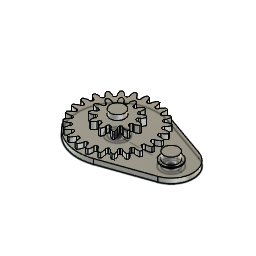
spur_gear_v2 (Autodesk Fusion 360 design; units mm, degrees)
part number: 2025-08-28-16-30-15-066
description: Spur Gear; Module: 3.0; Num Teeth: 24; Pressure Angle: 20.0; Backlash: 0.25 mm
part number: 2025-08-28-16-46-57-716
description: Spur Gear; Module: 3.0; Num Teeth: 12; Pressure Angle: 20.0; Backlash: 0.25 mm
part number: 2025-08-28-16-47-23-032
Autodesk Fusion 360 part; units mm, degrees
sketch "Sketch1" plane through (0, 0, 0) normal (0, 0, 1) x (1, 0, 0) in component "Spur Gear (24 teeth)"
  circle A0 centre (0, 0) radius 32.3492
  circle A1 centre (0, 0) radius 7.5
extrude "Extrude1" add sketch "Sketch1" along normal blind 5 makes body 1 in component "Spur Gear (24 teeth)"
sketch "Sketch2" plane through (0, 0, 0) normal (0, 0, 1) x (1, 0, 0) in component "Spur Gear (24 teeth)"
  spline S0 degree 5 poles (33.7244, -2.6568) (33.7396, -2.658) (33.77, -2.66) (33.8155, -2.6619) (33.8763, -2.6622) (33.9524, -2.6596) (34.0285, -2.6548) (34.1046, -2.6488) (34.1808, -2.642) (34.257, -2.6347) (34.3333, -2.6269) (34.4095, -2.6185) (34.4857, -2.6091) (34.5619, -2.5987) (34.6382, -2.5873) (34.7144, -2.5749) (34.7906, -2.5617) (34.8667, -2.5478) (34.9429, -2.5333) (35.019, -2.5183) (35.0952, -2.5027) (35.1712, -2.4864) (35.2473, -2.4696) (35.3234, -2.4521) (35.3994, -2.434) (35.4753, -2.4152) (35.5513, -2.3959) (35.6272, -2.376) (35.7031, -2.3556) (35.7789, -2.3347) (35.8547, -2.3132) (35.9304, -2.2912) (36.0062, -2.2688) (36.0818, -2.2458) (36.1575, -2.2223) (36.233, -2.1983) (36.3086, -2.1738) (36.384, -2.1488) (36.4595, -2.1233) (36.5349, -2.0974) (36.6102, -2.071) (36.6855, -2.0442) (36.7607, -2.0169) (36.8358, -1.9892) (36.911, -1.961) (36.986, -1.9324) (37.061, -1.9033) (37.1359, -1.8738) (37.2108, -1.8439) (37.2856, -1.8135) (37.3604, -1.7828) (37.435, -1.7516) (37.5097, -1.72) (37.5842, -1.688) (37.6587, -1.6556) (37.7331, -1.6227) (37.8075, -1.5895) (37.8818, -1.5559) (37.956, -1.5219) (38.0301, -1.4875) (38.1042, -1.4527) (38.1782, -1.4175) (38.2521, -1.3819) (38.3259, -1.346) (38.3997, -1.3096) (38.4734, -1.2729) (38.547, -1.2358) (38.6206, -1.1984) (38.694, -1.1606) (38.7674, -1.1224) (38.8407, -1.0838) (38.8993, -1.0527) (38.9432, -1.0292) (38.9724, -1.0134) (38.987, -1.0055) knots 0 0 0 0 0 0 0.01428571 0.02857143 0.04285714 0.05714286 0.07142857 0.08571429 0.1 0.11428571 0.12857143 0.14285714 0.15714286 0.17142857 0.18571429 0.2 0.21428571 0.22857143 0.24285714 0.25714286 0.27142857 0.28571429 0.3 0.31428571 0.32857143 0.34285714 0.35714286 0.37142857 0.38571429 0.4 0.41428571 0.42857143 0.44285714 0.45714286 0.47142857 0.48571429 0.5 0.51428571 0.52857143 0.54285714 0.55714286 0.57142857 0.58571429 0.6 0.61428571 0.62857143 0.64285714 0.65714286 0.67142857 0.68571429 0.7 0.71428571 0.72857143 0.74285714 0.75714286 0.77142857 0.78571429 0.8 0.81428571 0.82857143 0.84285714 0.85714286 0.87142857 0.88571429 0.9 0.91428571 0.92857143 0.94285714 0.95714286 0.97142857 0.98571429 1 1 1 1 1 1
  spline S1 degree 5 poles (33.7244, 2.6568) (33.7396, 2.658) (33.77, 2.66) (33.8155, 2.6619) (33.8763, 2.6622) (33.9524, 2.6596) (34.0285, 2.6548) (34.1046, 2.6488) (34.1808, 2.642) (34.257, 2.6347) (34.3333, 2.6269) (34.4095, 2.6185) (34.4857, 2.6091) (34.5619, 2.5987) (34.6382, 2.5873) (34.7144, 2.5749) (34.7906, 2.5617) (34.8667, 2.5478) (34.9429, 2.5333) (35.019, 2.5183) (35.0952, 2.5027) (35.1712, 2.4864) (35.2473, 2.4696) (35.3234, 2.4521) (35.3994, 2.434) (35.4753, 2.4152) (35.5513, 2.3959) (35.6272, 2.376) (35.7031, 2.3556) (35.7789, 2.3347) (35.8547, 2.3132) (35.9304, 2.2912) (36.0062, 2.2688) (36.0818, 2.2458) (36.1575, 2.2223) (36.233, 2.1983) (36.3086, 2.1738) (36.384, 2.1488) (36.4595, 2.1233) (36.5349, 2.0974) (36.6102, 2.071) (36.6855, 2.0442) (36.7607, 2.0169) (36.8358, 1.9892) (36.911, 1.961) (36.986, 1.9324) (37.061, 1.9033) (37.1359, 1.8738) (37.2108, 1.8439) (37.2856, 1.8135) (37.3604, 1.7828) (37.435, 1.7516) (37.5097, 1.72) (37.5842, 1.688) (37.6587, 1.6556) (37.7331, 1.6227) (37.8075, 1.5895) (37.8818, 1.5559) (37.956, 1.5219) (38.0301, 1.4875) (38.1042, 1.4527) (38.1782, 1.4175) (38.2521, 1.3819) (38.3259, 1.346) (38.3997, 1.3096) (38.4734, 1.2729) (38.547, 1.2358) (38.6206, 1.1984) (38.694, 1.1606) (38.7674, 1.1224) (38.8407, 1.0838) (38.8993, 1.0527) (38.9432, 1.0292) (38.9724, 1.0134) (38.987, 1.0055) knots 0 0 0 0 0 0 0.01428571 0.02857143 0.04285714 0.05714286 0.07142857 0.08571429 0.1 0.11428571 0.12857143 0.14285714 0.15714286 0.17142857 0.18571429 0.2 0.21428571 0.22857143 0.24285714 0.25714286 0.27142857 0.28571429 0.3 0.31428571 0.32857143 0.34285714 0.35714286 0.37142857 0.38571429 0.4 0.41428571 0.42857143 0.44285714 0.45714286 0.47142857 0.48571429 0.5 0.51428571 0.52857143 0.54285714 0.55714286 0.57142857 0.58571429 0.6 0.61428571 0.62857143 0.64285714 0.65714286 0.67142857 0.68571429 0.7 0.71428571 0.72857143 0.74285714 0.75714286 0.77142857 0.78571429 0.8 0.81428571 0.82857143 0.84285714 0.85714286 0.87142857 0.88571429 0.9 0.91428571 0.92857143 0.94285714 0.95714286 0.97142857 0.98571429 1 1 1 1 1 1
  arc A0 (38.987, -1.0055) -> (38.987, 1.0055) centre (0, 0) ccw
  line L0 (32.2393, -2.5406) -> (33.7244, -2.6568)
  line L1 (32.2393, 2.5406) -> (33.7244, 2.6568)
  line L2 (32.2393, -2.5406) -> (32.2393, 2.5406)
  point P0 (34.0955, -2.6493)
  point P1 (34.4689, -2.611)
  point P2 (34.8437, -2.552)
  point P3 (35.2195, -2.4757)
  point P4 (35.596, -2.3841)
  point P5 (35.973, -2.2785)
  point P6 (36.3504, -2.1599)
  point P7 (36.7278, -2.0288)
  point P8 (37.1053, -1.8858)
  point P9 (37.4826, -1.7314)
  point P10 (37.8595, -1.5659)
  point P11 (38.236, -1.3896)
  point P12 (38.6119, -1.2027)
  point P13 (34.0955, 2.6493)
  point P14 (34.4689, 2.611)
  point P15 (34.8437, 2.552)
  point P16 (35.2195, 2.4757)
  point P17 (35.596, 2.3841)
  point P18 (35.973, 2.2785)
  point P19 (36.3504, 2.1599)
  point P20 (36.7278, 2.0288)
  point P21 (37.1053, 1.8858)
  point P22 (37.4826, 1.7314)
  point P23 (37.8595, 1.5659)
  point P24 (38.236, 1.3896)
  point P25 (38.6119, 1.2027)
extrude "Extrude2" add sketch "Sketch2" along normal blind 5 bodies 1 in component "Spur Gear (24 teeth)"
fillet "Fillet1" radius 1.58 2 edges at (32.2492, -2.5414, 2.5) (32.2492, 2.5414, 2.5) on bodies 1 in component "Spur Gear (24 teeth)"
pattern_circular "C-Pattern1" count 24 over 360 about axis through (0, 0, 0) along (0, 0, 1) of "Extrude2", "Fillet1" in component "Spur Gear (24 teeth)"
sketch "Sketch3" plane through (0, 0, 0) normal (0, 0, 1) x (1, 0, 0) in component "Spur Gear (24 teeth)"
  circle A0 centre (0, 0) radius 36 construction
sketch "Sketch1 (2)" plane through (0, 0, 0) normal (0, 0, 1) x (1, 0, 0) in component "Spur Gear (12 teeth)"
  circle A0 centre (0, 0) radius 14.3492
  circle A1 centre (0, 0) radius 7.5
extrude "Extrude1'" add sketch "Sketch1 (2)" along normal blind 5 separate body makes body 2 in component "Spur Gear (12 teeth)"
sketch "Sketch2 (2)" plane through (0, 0, 0) normal (0, 0, 1) x (1, 0, 0) in component "Spur Gear (12 teeth)"
  spline S0 degree 5 poles (16.7434, -2.3993) (16.7555, -2.4011) (16.7797, -2.4041) (16.816, -2.4076) (16.8646, -2.4099) (16.9256, -2.4099) (16.9867, -2.4077) (17.048, -2.4042) (17.1093, -2.3999) (17.1707, -2.3952) (17.2321, -2.3899) (17.2936, -2.3839) (17.3551, -2.377) (17.4166, -2.369) (17.4782, -2.3599) (17.5398, -2.3498) (17.6015, -2.3389) (17.6631, -2.3273) (17.7248, -2.3151) (17.7864, -2.3023) (17.8481, -2.2889) (17.9097, -2.2748) (17.9713, -2.2601) (18.0329, -2.2447) (18.0945, -2.2286) (18.1561, -2.2119) (18.2176, -2.1946) (18.2792, -2.1767) (18.3407, -2.1582) (18.4021, -2.1392) (18.4635, -2.1196) (18.5249, -2.0995) (18.5863, -2.0788) (18.6476, -2.0576) (18.7089, -2.0358) (18.7701, -2.0135) (18.8312, -1.9906) (18.8923, -1.9673) (18.9534, -1.9434) (19.0144, -1.9191) (19.0753, -1.8942) (19.1362, -1.8689) (19.197, -1.8431) (19.2578, -1.8167) (19.3185, -1.7899) (19.3791, -1.7626) (19.4396, -1.7349) (19.5001, -1.7066) (19.5605, -1.6779) (19.6208, -1.6488) (19.681, -1.6192) (19.7412, -1.5891) (19.8013, -1.5586) (19.8612, -1.5276) (19.9211, -1.4962) (19.981, -1.4644) (20.0407, -1.4321) (20.1003, -1.3994) (20.1598, -1.3662) (20.2193, -1.3327) (20.2786, -1.2986) (20.3379, -1.2642) (20.397, -1.2294) (20.456, -1.1941) (20.515, -1.1584) (20.5738, -1.1223) (20.6325, -1.0858) (20.6911, -1.0489) (20.7496, -1.0116) (20.808, -0.9739) (20.8663, -0.9357) (20.9128, -0.9049) (20.9477, -0.8816) (20.9709, -0.866) (20.9825, -0.8582) knots 0 0 0 0 0 0 0.01428571 0.02857143 0.04285714 0.05714286 0.07142857 0.08571429 0.1 0.11428571 0.12857143 0.14285714 0.15714286 0.17142857 0.18571429 0.2 0.21428571 0.22857143 0.24285714 0.25714286 0.27142857 0.28571429 0.3 0.31428571 0.32857143 0.34285714 0.35714286 0.37142857 0.38571429 0.4 0.41428571 0.42857143 0.44285714 0.45714286 0.47142857 0.48571429 0.5 0.51428571 0.52857143 0.54285714 0.55714286 0.57142857 0.58571429 0.6 0.61428571 0.62857143 0.64285714 0.65714286 0.67142857 0.68571429 0.7 0.71428571 0.72857143 0.74285714 0.75714286 0.77142857 0.78571429 0.8 0.81428571 0.82857143 0.84285714 0.85714286 0.87142857 0.88571429 0.9 0.91428571 0.92857143 0.94285714 0.95714286 0.97142857 0.98571429 1 1 1 1 1 1
  spline S1 degree 5 poles (16.7434, 2.3993) (16.7555, 2.4011) (16.7797, 2.4041) (16.816, 2.4076) (16.8646, 2.4099) (16.9256, 2.4099) (16.9867, 2.4077) (17.048, 2.4042) (17.1093, 2.3999) (17.1707, 2.3952) (17.2321, 2.3899) (17.2936, 2.3839) (17.3551, 2.377) (17.4166, 2.369) (17.4782, 2.3599) (17.5398, 2.3498) (17.6015, 2.3389) (17.6631, 2.3273) (17.7248, 2.3151) (17.7864, 2.3023) (17.8481, 2.2889) (17.9097, 2.2748) (17.9713, 2.2601) (18.0329, 2.2447) (18.0945, 2.2286) (18.1561, 2.2119) (18.2176, 2.1946) (18.2792, 2.1767) (18.3407, 2.1582) (18.4021, 2.1392) (18.4635, 2.1196) (18.5249, 2.0995) (18.5863, 2.0788) (18.6476, 2.0576) (18.7089, 2.0358) (18.7701, 2.0135) (18.8312, 1.9906) (18.8923, 1.9673) (18.9534, 1.9434) (19.0144, 1.9191) (19.0753, 1.8942) (19.1362, 1.8689) (19.197, 1.8431) (19.2578, 1.8167) (19.3185, 1.7899) (19.3791, 1.7626) (19.4396, 1.7349) (19.5001, 1.7066) (19.5605, 1.6779) (19.6208, 1.6488) (19.681, 1.6192) (19.7412, 1.5891) (19.8013, 1.5586) (19.8612, 1.5276) (19.9211, 1.4962) (19.981, 1.4644) (20.0407, 1.4321) (20.1003, 1.3994) (20.1598, 1.3662) (20.2193, 1.3327) (20.2786, 1.2986) (20.3379, 1.2642) (20.397, 1.2294) (20.456, 1.1941) (20.515, 1.1584) (20.5738, 1.1223) (20.6325, 1.0858) (20.6911, 1.0489) (20.7496, 1.0116) (20.808, 0.9739) (20.8663, 0.9357) (20.9128, 0.9049) (20.9477, 0.8816) (20.9709, 0.866) (20.9825, 0.8582) knots 0 0 0 0 0 0 0.01428571 0.02857143 0.04285714 0.05714286 0.07142857 0.08571429 0.1 0.11428571 0.12857143 0.14285714 0.15714286 0.17142857 0.18571429 0.2 0.21428571 0.22857143 0.24285714 0.25714286 0.27142857 0.28571429 0.3 0.31428571 0.32857143 0.34285714 0.35714286 0.37142857 0.38571429 0.4 0.41428571 0.42857143 0.44285714 0.45714286 0.47142857 0.48571429 0.5 0.51428571 0.52857143 0.54285714 0.55714286 0.57142857 0.58571429 0.6 0.61428571 0.62857143 0.64285714 0.65714286 0.67142857 0.68571429 0.7 0.71428571 0.72857143 0.74285714 0.75714286 0.77142857 0.78571429 0.8 0.81428571 0.82857143 0.84285714 0.85714286 0.87142857 0.88571429 0.9 0.91428571 0.92857143 0.94285714 0.95714286 0.97142857 0.98571429 1 1 1 1 1 1
  arc A0 (20.9825, -0.8582) -> (20.9825, 0.8582) centre (0, 0) ccw
  line L0 (14.1942, -2.0355) -> (16.7434, -2.3993)
  line L1 (14.1942, 2.0355) -> (16.7434, 2.3993)
  line L2 (14.1942, -2.0355) -> (14.1942, 2.0355)
  point P0 (17.0374, -2.4046)
  point P1 (17.3356, -2.379)
  point P2 (17.6364, -2.3323)
  point P3 (17.939, -2.2677)
  point P4 (18.2429, -2.1871)
  point P5 (18.5478, -2.0917)
  point P6 (18.8533, -1.9821)
  point P7 (19.1591, -1.8591)
  point P8 (19.4648, -1.7231)
  point P9 (19.7701, -1.5744)
  point P10 (20.0748, -1.4133)
  point P11 (20.3787, -1.2401)
  point P12 (20.6813, -1.055)
  point P13 (17.0374, 2.4046)
  point P14 (17.3356, 2.379)
  point P15 (17.6364, 2.3323)
  point P16 (17.939, 2.2677)
  point P17 (18.2429, 2.1871)
  point P18 (18.5478, 2.0917)
  point P19 (18.8533, 1.9821)
  point P20 (19.1591, 1.8591)
  point P21 (19.4648, 1.7231)
  point P22 (19.7701, 1.5744)
  point P23 (20.0748, 1.4133)
  point P24 (20.3787, 1.2401)
  point P25 (20.6813, 1.055)
extrude "Extrude2'" add sketch "Sketch2 (2)" along normal blind 5 bodies 2 in component "Spur Gear (12 teeth)"
fillet "Fillet1'" radius 1.58 2 edges at (14.2039, -2.0368, 2.5) (14.2039, 2.0368, 2.5) on bodies 2 in component "Spur Gear (12 teeth)"
pattern_circular "C-Pattern1'" count 12 over 360 about axis through (0, 0, 0) along (0, 0, 1) of "Extrude2'", "Fillet1'" in component "Spur Gear (12 teeth)"
sketch "Sketch3 (2)" plane through (0, 0, 0) normal (0, 0, 1) x (1, 0, 0) in component "Spur Gear (12 teeth)"
  circle A0 centre (0, 0) radius 18 construction
move_body "Move1" bodies 1 to x (1, 0, 0) y (0, 1, 0) z (0, 0, 1) at (0, 80, 0) in component "Spur Gear (24 teeth)"
move_body "Move1'" bodies 2 to x (1, 0, 0) y (0, 1, 0) z (0, 0, 1) at (0, -80, 0) in component "Spur Gear (12 teeth)"
sketch "Sketch1 (3)" plane through (0, 0, 0) normal (0, 0, 1) x (1, 0, 0)
  line L0 (0, 0) -> (54.25, 0) construction
  line L1 (13.2719, -37.734) -> (61.5495, -20.7537)
  line L2 (13.2719, 37.734) -> (61.5495, 20.7537)
  arc A0 (61.5495, -20.7537) -> (61.5495, 20.7537) centre (54.25, 0) ccw
  arc A1 (13.2719, 37.734) -> (13.2719, -37.734) centre (0, 0) ccw
  circle A2 centre (0, 0) radius 7.4
  circle A3 centre (54.25, 0) radius 7.4
  circle A4 centre (0, 0) radius 10
  circle A5 centre (54.25, 0) radius 10
  dimension "d17" = 80
  dimension "d18" = 54.25
  dimension "d19" = 44
  dimension "d20" = 14.8
  dimension "d21" = 14.8
  dimension "d22" = 20
  dimension "d23" = 20
  constraint coincident L0.start A1.centre
  constraint horizontal L0
  constraint coincident L0.end A0.centre
  constraint tangent L1 A1
  constraint tangent L1 A0
  constraint tangent L2 A0
  constraint tangent L2 A1
  constraint concentric A0 A3
  constraint concentric A1 A4
  constraint concentric A0 A5
  measures "d17" diameter of A1
  measures "d18" distance of L0.start L0.end
  measures "d19" diameter of A0
  measures "d20" diameter of A2
  measures "d21" diameter of A3
  measures "d22" diameter of A4
  measures "d23" diameter of A5
extrude "Extrude1''" add sketch "Sketch1 (3)" along normal blind 5 separate body contours L1 L2 A0 A1 makes body 3
extrude "Extrude2''" add sketch "Sketch1 (3)" along normal blind 6 contours A4 bodies 3
extrude "Extrude3" add sketch "Sketch1 (3)" along normal blind 13 contours A2 bodies 3
extrude "Extrude4" add sketch "Sketch1 (3)" along normal up to surface (13 mm away) separate body contours A3 makes body 4
extrude "Extrude5" add sketch "Sketch1 (3)" along normal up to surface (6 mm away) contours A5 bodies 3 4
move_body "Move2" bodies 2 to x (1, 0, 0) y (0, 1, 0) z (0, 0, 1) at (0, 10, 0) in component "Spur Gear (12 teeth)"
move_body "Move2'" bodies 1 to x (1, 0, 0) y (0, 1, 0) z (0, 0, 1) at (0, 10, 0) in component "Spur Gear (24 teeth)"
move_body "Move3" bodies 1 to x (1, 0, 0) y (0, 1, 0) z (0, 0, 1) at (0, -8, 0) in component "Spur Gear (24 teeth)"
move_body "Move3'" bodies 2 to x (1, 0, 0) y (0, 1, 0) z (0, 0, 1) at (0, 5, 0) in component "Spur Gear (12 teeth)"
move_body "Move4" bodies 2 to x (0.707107, -0.707107, 0) y (0.707107, 0.707107, 0) z (0, 0, 1) at (15.8895, 38.3605, 0) in component "Spur Gear (12 teeth)"
move_body "Move5" bodies 2 to x (1, 0, 0) y (0, 1, 0) z (0, 0, 1) at (40, 0, 30) in component "Spur Gear (12 teeth)"
combine "Combine1" operation add target body 1 tool bodies 2 body 2 seen with x (-0.751235, -0.660035, 0) y (0.660035, -0.751235, 0) z (0, 0, 1) at (12.4751, 82.8421, -28) in component "Spur Gear (24 teeth)"
extrude "Extrude6" add 1 faces at (-2.2558, -0.556, 13) along direction (0, 0, 1) blind 10 on bodies 3 bodies 3
extrude "Extrude3'" add 1 faces at (-12.0022, 82.7756, 7) along direction (0, 0, 1) blind 5 on bodies 1 bodies 1 in component "Spur Gear (24 teeth)"
component "Spur Gear (12 teeth)" placed x (0.148017, -0.988985, 0) y (0.988985, 0.148017, 0) z (0, 0, 1) at (6.0482, 10.9433, -22)
component "Spur Gear (24 teeth)" placed x (-0.454282, 0.890858, 0) y (-0.890858, -0.454282, 0) z (0, 0, 1) at (73.0504, 37.2511, 6)
